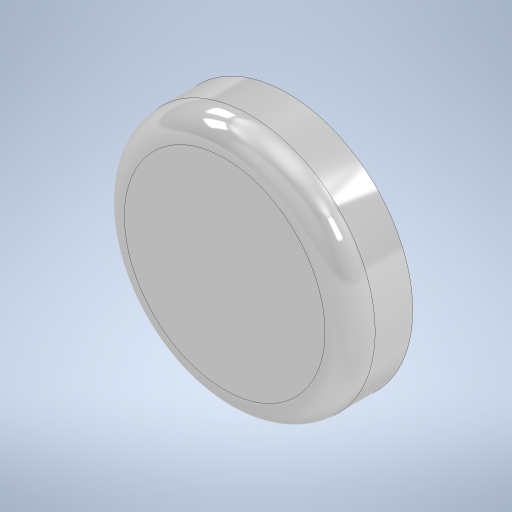
# Autodesk Inventor part: Buttonx20
Saved by Autodesk Inventor 2024 (Build 280153000, 153)
## iProperties
Created: 2023-09-15
Part Number: Buttonx20
Material: 玻璃
Document SubType Name: Modeling
Designer: nicx5
Density: 2.18 g/cm^3
Appearance: 铝 - 抛光
Author: nicx5
Autodesk Inventor part; units mm, degrees
ref_plane "YZ Plane" through (0, 0, 0) normal (1, 0, 0) x (0, 1, 0)
ref_plane "XZ Plane" through (0, 0, 0) normal (0, 1, 0) x (-1, 0, 0)
ref_plane "XY Plane" through (0, 0, 0) normal (0, 0, 1) x (1, 0, 0)
sketch "草图1" plane through (0, 0, 0) normal (0, 1, 0) x (-1, 0, 0)
  circle A0 centre (0, 0) radius 10
  dimension "d0" = 20
  constraints: 1 centre point
  measures "d0" diameter of A0
extrude "拉伸1" add sketch "草图1" against normal blind 5
fillet "圆角1" radius 2 1 edges at (10, 0, 0)
shell "抽壳1" thickness 1.5 removed faces 1 at (1.182, -5, 3.1167)
move or copy body "旋转1" bodies to move or copy 1 copy no rotation origin (0, 0, 0) rotation axis (1, 0, 0) rotation angle 90 translate (0, -1.5, 1.5)
